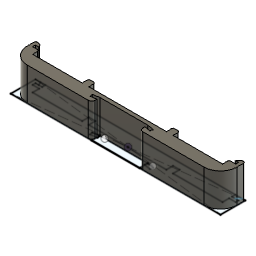
socket-din-rail-mount v1 (Autodesk Fusion 360 design; units mm, degrees)
Autodesk Fusion 360 part; units mm, degrees
sketch "Sketch1" plane through (0, 0, 0) normal (0, 1, 0) x (1, 0, 0)
  line L0 (63.5, 7.5) -> (-63.5, 7.5)
  line L1 (-63.5, 7.5) -> (-63.5, -7.5)
  line L2 (-63.5, -7.5) -> (63.5, -7.5)
  line L3 (63.5, -7.5) -> (63.5, 7.5)
  line L4 (63.5, 7.5) -> (-63.5, -7.5) construction
  line L5 (-63.5, 7.5) -> (63.5, -7.5) construction
  line L6 (0, -7.5) -> (-14.5, -7.5) construction
  line L7 (-14.5, -7.5) -> (14.5, -7.5)
  line L8 (14.5, -7.5) -> (14.5, -2.5)
  line L9 (14.5, -2.5) -> (-14.5, -2.5)
  line L10 (-14.5, -2.5) -> (-14.5, -7.5)
  line L11 (-14.5, -2.5) -> (-18.4392, -3.1946)
  line L12 (-14.5, -2.5) -> (-11.5456, -2.5) construction
  line L13 (-14.5, -2.5) -> (-18.4392, -3.1946)
  line L14 (-18.4392, -3.1946) -> (-18.1353, -4.918)
  line L15 (-18.1353, -4.918) -> (-14.1961, -4.2234)
  line L16 (-14.1961, -4.2234) -> (-14.5, -2.5)
  line L17 (14.5, -2.5) -> (18.4392, -3.1946)
  line L18 (14.5, -2.5) -> (17.5, -2.5) construction
  line L19 (14.5, -2.5) -> (18.4392, -3.1946)
  line L20 (18.4392, -3.1946) -> (18.1353, -4.918)
  line L21 (18.1353, -4.918) -> (14.1961, -4.2234)
  line L22 (14.1961, -4.2234) -> (14.5, -2.5)
  line L23 (-63.5, 7.5) -> (-57.5, 7.5) construction
  line L24 (-57.5, 7.5) -> (-57.5, 5.5)
  line L25 (-57.5, 5.5) -> (-61.5, 5.5)
  line L26 (-61.5, 5.5) -> (-61.5, 3.75)
  line L27 (61.5, 3.7349) -> (61.5066, 5.4848)
  line L28 (61.5066, 5.4848) -> (57.5067, 5.5)
  line L29 (57.5067, 5.5) -> (57.5067, 7.5)
  line L30 (-61.5, 3.75) -> (-57.5, 3.75)
  line L31 (-57.5, 3.75) -> (-57.5, -0.25)
  line L32 (-57.5, -0.25) -> (-27.5, -0.25)
  line L33 (-27.5, -0.25) -> (-27.5, 3.75)
  line L34 (-27.5, 3.75) -> (-23.5, 3.75)
  line L35 (-23.5, 3.75) -> (-23.5, -0.25)
  line L36 (-23.5, -0.25) -> (23.5, -0.25)
  line L37 (23.5, -0.25) -> (23.5, 3.75)
  line L38 (23.5, 3.75) -> (27.5, 3.75)
  line L39 (27.5, 3.75) -> (27.5, -0.25)
  line L40 (27.5, -0.25) -> (57.5, -0.25)
  line L41 (57.5, -0.25) -> (57.5, 3.75)
  line L42 (57.5, 3.75) -> (61.5, 3.7349)
  line L43 (-61.5, 5.5) -> (-59.5, 5.5) construction
  line L44 (-60.5, 7.5) -> (-59.5, 5.5)
  line L45 (61.5066, 5.4848) -> (59.5066, 5.4924) construction
  line L46 (61.5452, 7.5) -> (59.5066, 5.4924)
  dimension "d1" = 127
  dimension "d2" = 15
  dimension "d3" = 14.5
  dimension "d5" = 29
  dimension "d6" = 5
  dimension "d7" = 190
  dimension "d8" = 4
  dimension "d9" = 1.75
  dimension "d10" = 4
  dimension "d11" = 190
  dimension "d12" = 1.75
  dimension "d15" = 6
  dimension "d16" = 2
  dimension "d17" = 4
  dimension "d18" = 1.75
  dimension "d19" = 123
  dimension "d20" = 1.75
  dimension "d21" = 4
  dimension "d22" = 2
  dimension "d23" = 4
  dimension "d24" = 4
  dimension "d25" = 30
  dimension "d26" = 4
  dimension "d27" = 4
  dimension "d28" = 47
  dimension "d29" = 4
  dimension "d30" = 4
  dimension "d31" = 4
  dimension "d32" = 30
  dimension "d33" = 4
  dimension "d38" = 89.783
  constraint horizontal L0
  constraint perpendicular L0 L1
  constraint parallel L0 L2
  constraint parallel L1 L3
  constraint coincident L4 origin
  constraint coincident L5 origin
  constraint horizontal L6
  constraint midpoint L2 L6.start
  constraint horizontal L7
  constraint vertical L8
  constraint horizontal L9
  constraint vertical L10
  constraint horizontal L12
  constraint perpendicular L13 L14
  constraint parallel L13 L15
  constraint parallel L14 L16
  constraint horizontal L18
  constraint perpendicular L19 L20
  constraint parallel L19 L21
  constraint parallel L20 L22
  constraint perpendicular L1 L23
  constraint perpendicular L2 L24
  constraint horizontal L25
  constraint perpendicular L25 L26
  constraint perpendicular L27 L28
  constraint vertical L29
  constraint perpendicular L26 L30
  constraint vertical L31
  constraint perpendicular L31 L32
  constraint perpendicular L32 L33
  constraint perpendicular L33 L34
  constraint perpendicular L34 L35
  constraint perpendicular L35 L36
  constraint vertical L37
  constraint perpendicular L37 L38
  constraint vertical L39
  constraint perpendicular L37 L40
  constraint perpendicular L40 L41
  constraint perpendicular L27 L42
  constraint coincident L0 L29.end
  constraint midpoint L25 L43.end
  constraint midpoint L23 L44.start
  constraint midpoint L28 L45.end
  constraint coincident L0 L46.start
  measures "d1" distance of L1.end L2.end
  measures "d2" distance of L0.end L1.end
  measures "d3" distance of L6.start L6.end
  measures "d5" distance of L6.end L7.end
  measures "d6" distance of L6.end L9.end
  measures "d8" distance of L9.end L11.end
  measures "d9" distance of L9.end L15.end
  measures "d10" distance of L8.end L17.end
  measures "d12" distance of L8.end L21.end
  measures "d15" distance of L0.end L23.end
  measures "d16" distance of L23.end L24.end
  measures "d17" distance of L24.end L25.end
  measures "d18" distance of L25.end L26.end
  measures "d19" distance of L26.end L27.start
  measures "d20" distance of L27.start L27.end
  measures "d21" distance of L27.end L28.end
  measures "d22" distance of L28.end L29.end
  measures "d23" distance of L26.end L30.end
  measures "d24" distance of L30.end L31.end
  measures "d25" distance of L31.end L32.end
  measures "d26" distance of L32.end L33.end
  measures "d27" distance of L33.end L34.end
  measures "d28" distance of L35.end L36.end
  measures "d29" distance of L36.end L37.end
  measures "d30" distance of L37.end L38.end
  measures "d31" distance of L38.end L39.end
  measures "d32" distance of L39.end L40.end
  measures "d33" distance of L40.end L41.end
  measures "d38" angle of L31 L42
extrude "Extrude3" add sketch "Sketch1" along normal blind 20 contours L0 L1 L2 L3 L8 L9 L10 L11 L13 L14 L15 L17 L19 L20 L21 L25 L26 L27 L28 L30 L31 L32 L33 L34 L35 L36 L37 L38 L39 L40 L41 L42 L44 L46
fillet "Fillet1" radius 10 2 edges at (-63.5, 10, 7.5) (63.5, 10, 7.5)
fillet "Fillet2" radius 1 6 edges at (-57.5, 10, -3.75) (-27.5, 10, -3.75) (-23.5, 10, -3.75) (23.5, 10, -3.75) (27.5, 10, -3.75) (57.5, 10, -3.75)
fillet "Fillet3" radius 1 2 edges at (-63.5, 10, -7.5) (63.5, 10, -7.5)
fillet "Fillet4" radius 2 2 edges at (-60.5, 10, -7.5) (61.5452, 10, -7.5)
fillet "Fillet5" radius 2 2 edges at (-14.5, 10, 7.5) (14.5, 10, 7.5)
equation "d3 = ( 35 / 2 ) * 1 mm - 3 mm"
